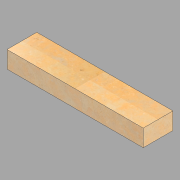
# Autodesk Inventor part: Sconce_Backer_4
Saved by Autodesk Inventor 2022.1 (Build 261234020, 234B)
## iProperties
Created: 2021-12-03
Part Number: Sconce_Backer_4
Material: Limestone
Document SubType Name: Modeling
Designer: awelt
Density: 2.6 g/cm^3
Appearance: Amber Select
Mass: 16105.2 g
Surface Area: 2758.06 cm^2
Volume: 6194.31 cm^3
Author: awelt
Autodesk Inventor part; units mm, degrees
ref_plane "YZ Plane" through (0, 0, 0) normal (1, 0, 0) x (0, 1, 0)
ref_plane "XZ Plane" through (0, 0, 0) normal (0, 1, 0) x (-1, 0, 0)
ref_plane "XY Plane" through (0, 0, 0) normal (0, 0, 1) x (1, 0, 0)
sketch "Sketch1" plane through (0, 0, 0) normal (0, 1, 0) x (-1, 0, 0)
  line L0 (304.8, -66.675) -> (-304.8, -66.675)
  line L1 (-304.8, -66.675) -> (-304.8, 66.675)
  line L2 (-304.8, 66.675) -> (304.8, 66.675)
  line L3 (304.8, 66.675) -> (304.8, -66.675)
  line L4 (304.8, -66.675) -> (-304.8, 66.675) construction
  line L5 (-304.8, -66.675) -> (304.8, 66.675) construction
  point P0 (0, 0)
  dimension "d0" = 609.6
  dimension "d1" = 133.35
  constraints: 12 end point, 2 midpoint, 2 parallel, 1 horizontal, 1 perpendicular
  measures "d0" distance of L1.end L2.end
  measures "d1" distance of L0.end L1.end
extrude "Extrusion1" add sketch "Sketch1" along normal blind 76.2
body "Solid1"
